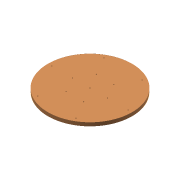
# Autodesk Inventor part: bpSparJig
Saved by Autodesk Inventor 2016 (Build 200138000, 138)
## iProperties
Created: 2015-05-20
Part Number: bpSparJig
Material: Wood (Cherry)
Document SubType Name: Modeling
Designer: Dave
Mass: 1169.13 g
Surface Area: 1704.61 cm^2
Volume: 1855.77 cm^3
Density: 0.63 g/cm^3
Appearance: Cherry - Natural Low Gloss
Author: Dave
Autodesk Inventor part; units mm, degrees
ref_plane "YZ Plane" through (0, 0, 0) normal (1, 0, 0) x (0, 1, 0)
ref_plane "XZ Plane" through (0, 0, 0) normal (0, 1, 0) x (-1, 0, 0)
ref_plane "XY Plane" through (0, 0, 0) normal (0, 0, 1) x (1, 0, 0)
sketch "Sketch1" plane through (0, 0, 0) normal (0, 1, 0) x (-1, 0, 0)
  circle A0 centre (0.7015, 0) radius 305
  point P0 (0, 0)
  dimension "d0" = 610
  constraints: 1 centre point
  measures "d0" diameter of A0
extrude "Extrusion1" add sketch "Sketch1" along normal blind 25.4
sketch "Sketch2" plane through (-0.7015, 25.4, 0) normal (0, 1, 0) x (1, 0, 0)
  circle A0 centre (0, 0) radius 305 projected
  circle A1 centre (0, 0) radius 4.5
  circle A2 centre (127, 0) radius 4.5
  circle A3 centre (277, 0) radius 4.5
  dimension "d3" = 127
  dimension "d4" = 150
  dimension "d15" = 9
  dimension "d16" = 9
  dimension "d17" = 9
  constraints: 3 centre point, 2 coincident
  measures "d3" distance of A2.centre A0.centre
  measures "d4" distance of A3.centre A2.centre
  measures "d15" diameter of A1
  measures "d16" diameter of A2
  measures "d17" diameter of A3
hole "Hole1" at (-0.7015, 25.4, 0) at (126.2985, 25.4, 0) at (276.2985, 25.4, 0) direction (0, -1, 0) diameter 6.35 end through all
pattern_circular "Circular Pattern1" count 6 over 360 about axis through (-0.7015, -837.6441, 0) along (0, 1, 0) of "Hole1"
body "Solid1"
